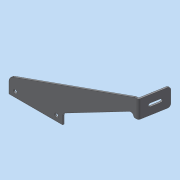
# Autodesk Inventor part: 0 零件
Saved by Autodesk Inventor 2020 (Build 240168000, 168)
## iProperties
Created: 2020-11-03
Part Number: 0 零件
Material: 一般
Document SubType Name: Modeling
Designer: p2013
Density: 1 g/cm^3
Appearance: 預設
Author: p2013
Autodesk Inventor part; units mm, degrees
ref_plane "YZ Plane" through (0, 0, 0) normal (1, 0, 0) x (0, 1, 0)
ref_plane "XZ Plane" through (0, 0, 0) normal (0, 1, 0) x (-1, 0, 0)
ref_plane "XY Plane" through (0, 0, 0) normal (0, 0, 1) x (1, 0, 0)
sketch "草圖1" plane through (0, 0, 0) normal (0, 0, 1) x (1, 0, 0)
  line L0 (0, 0) -> (-7.8042, 0) construction
  line L1 (0, 0) -> (0, -16.694) construction
  line L2 (0, 0) -> (0, 26)
  line L3 (310, 145) -> (310, 102)
  line L4 (130, 18.5892) -> (130, 0)
  line L5 (130, 0) -> (0, 0)
  line L6 (310, 145) -> (368, 145)
  line L7 (375, 138) -> (375, 109)
  line L8 (368, 102) -> (310, 102)
  line L9 (332, 127.5) -> (354, 127.5)
  arc A0 (354, 119.5) -> (354, 127.5) centre (354, 123.5) ccw
  line L10 (354, 119.5) -> (332, 119.5)
  arc A1 (332, 127.5) -> (332, 119.5) centre (332, 123.5) ccw
  circle A2 centre (15, 12.5) radius 4.5
  circle A3 centre (115, 12.5) radius 4.5
  line L11 (15, 12.5) -> (115, 12.5) construction
  arc A4 (10.0507, 40.16) -> (0, 26) centre (15, 26) ccw
  line L12 (9.9762, 40.1337) -> (303.3752, 144.4225)
  line L13 (306.7244, 145) -> (310, 145)
  line L14 (310, 102) -> (305, 102)
  line L15 (291.9625, 109.2052) -> (135.372, 27.4539)
  arc A5 (375, 138) -> (368, 145) centre (368, 138) ccw
  arc A6 (368, 102) -> (375, 109) centre (368, 109) ccw
  arc A7 (302.0606, 104.4) -> (305, 102) centre (305, 105) ccw
  arc A8 (302.0606, 104.4) -> (291.9625, 109.2052) centre (295.202, 103) ccw
  arc A9 (306.7244, 145) -> (303.3752, 144.4225) centre (306.7244, 135) ccw
  arc A10 (135.372, 27.4539) -> (130, 18.5892) centre (140, 18.5892) ccw
  point P0 (130, 34.6822)
  point P1 (375, 145)
  point P2 (375, 102)
  point P3 (65, 12.5)
  point P4 (65, 0)
  point P5 (130, 24.6493)
  point P6 (305, 145)
  point P7 (305, 102)
  point P8 (305, 116.0118)
  dimension "d0" = 130
  dimension "d1" = 145
  dimension "d2" = 43
  dimension "d3" = 65
  dimension "d4" = 8
  dimension "d5" = 30
  dimension "d7" = 18
  dimension "d8" = 310
  dimension "d14" = 12.5
  dimension "d15" = 100
  dimension "d16" = 9
  dimension "d17" = 21.5
  dimension "d20" = 15
  dimension "d21" = 26
  dimension "d23" = 5
  dimension "d24" = 7
  dimension "d26" = 3
  dimension "d28" = 35
  dimension "d29" = 7
  dimension "d30" = 5
  dimension "d31" = 10
  dimension "d32" = 10
  dimension "d33" = 8
  constraints: 33 end point, 19 point on circle, 17 tangent, 11 centre point, 11 point on line, 6 horizontal, 3 parallel, 3 perpendicular, 3 vertical alignment, 2 equal radius, 2 midpoint, 2 vertical, 1 horizontal alignment
  measures "d0" distance between parallel lines of L4 L2
  measures "d1" distance from line of L3.start L5
  measures "d2" distance between parallel lines of L6 L8
  measures "d3" distance between parallel lines of L7 L3
  measures "d4" distance between parallel lines of L10 L9
  measures "d7" distance edge to line of A1 L3
  measures "d8" distance between parallel lines of L3 L2
  measures "d14" distance from line of L5 L11.start
  measures "d15" distance of L11.end L11.start
  measures "d16" diameter of A2
  measures "d17" distance from line of L6 A0.centre
  measures "d20" radius of A4
  measures "d21" distance of L0.start L2.end
  measures "d23" distance of point (305, 145) L3.start
  measures "d24" radius of A5
  measures "d26" radius of A7
  measures "d28" distance edge to line of A8 L13
  measures "d29" radius of A8
  measures "d30" distance of L3.end L14.end
  measures "d31" radius of A9
  measures "d32" radius of A10
  measures "d33" angle of L15 L12
extrude "擠出1" add sketch "草圖1" along normal blind 3.5
bend part "折彎零件1" radius 0.5 angle 80 line through (310, 145, 0) along (0, -1, 0) centre toward (0, 0, -1) moving side (1, 0, 0) both sides no
